Autodesk Fusion 360 part; units mm, degrees
(part 4 of 10)
sketch "草图11 (10)" plane through (0, 0, 36) normal (0, 0, 1) x (1, 0, 0) in component "LS_RemovableGrate"
  line L0 (60.3, 210) -> (159.7, 210)
  line L1 (159.7, 210) -> (159.7, 214)
  line L2 (159.7, 214) -> (60.3, 214)
  line L3 (60.3, 214) -> (60.3, 210)
  dimension "d1492" = 210
  dimension "d1493" = 99.4
  dimension "d1494" = 4
  constraint horizontal L0
  constraint vertical L1
  constraint horizontal L2
  constraint vertical L3
  measures "d1492" vertical distance of origin L0.start
  measures "d1493" horizontal distance of L0.start L0.end
  measures "d1494" vertical distance of L0.end L1.end
extrude "Drain slot 10''''" cut sketch "草图11 (10)" along normal blind 4 bodies 26 in component "LS_RemovableGrate"
ref_plane "工作平面12" through (0, 0, 36) normal (0, 0, 1) x (1, 0, 0) in component "LS_RemovableGrate"
sketch "草图12 (10)" plane through (0, 0, 36) normal (0, 0, 1) x (1, 0, 0) in component "LS_RemovableGrate"
  line L0 (60.3, 200) -> (159.7, 200)
  line L1 (159.7, 200) -> (159.7, 204)
  line L2 (159.7, 204) -> (60.3, 204)
  line L3 (60.3, 204) -> (60.3, 200)
  dimension "d1500" = 200
  dimension "d1501" = 99.4
  dimension "d1502" = 4
  constraint horizontal L0
  constraint vertical L1
  constraint horizontal L2
  constraint vertical L3
  measures "d1500" vertical distance of origin L0.start
  measures "d1501" horizontal distance of L0.start L0.end
  measures "d1502" vertical distance of L0.end L1.end
extrude "Drain slot 11''''" cut sketch "草图12 (10)" along normal blind 4 bodies 26 in component "LS_RemovableGrate"
ref_plane "工作平面13" through (0, 0, 36) normal (0, 0, 1) x (1, 0, 0) in component "LS_RemovableGrate"
sketch "草图13 (10)" plane through (0, 0, 36) normal (0, 0, 1) x (1, 0, 0) in component "LS_RemovableGrate"
  line L0 (60.3, 190) -> (159.7, 190)
  line L1 (159.7, 190) -> (159.7, 194)
  line L2 (159.7, 194) -> (60.3, 194)
  line L3 (60.3, 194) -> (60.3, 190)
  dimension "d1508" = 190
  dimension "d1509" = 99.4
  dimension "d1510" = 4
  constraint horizontal L0
  constraint vertical L1
  constraint horizontal L2
  constraint vertical L3
  measures "d1508" vertical distance of origin L0.start
  measures "d1509" horizontal distance of L0.start L0.end
  measures "d1510" vertical distance of L0.end L1.end
extrude "Drain slot 12''" cut sketch "草图13 (10)" along normal blind 4 bodies 26 in component "LS_RemovableGrate"
ref_plane "工作平面14" through (0, 0, 36) normal (0, 0, 1) x (1, 0, 0) in component "LS_RemovableGrate"
sketch "草图14 (8)" plane through (0, 0, 36) normal (0, 0, 1) x (1, 0, 0) in component "LS_RemovableGrate"
  line L0 (60.3, 180) -> (159.7, 180)
  line L1 (159.7, 180) -> (159.7, 184)
  line L2 (159.7, 184) -> (60.3, 184)
  line L3 (60.3, 184) -> (60.3, 180)
  dimension "d1516" = 180
  dimension "d1517" = 99.4
  dimension "d1518" = 4
  constraint horizontal L0
  constraint vertical L1
  constraint horizontal L2
  constraint vertical L3
  measures "d1516" vertical distance of origin L0.start
  measures "d1517" horizontal distance of L0.start L0.end
  measures "d1518" vertical distance of L0.end L1.end
extrude "Drain slot 13''" cut sketch "草图14 (8)" along normal blind 4 bodies 26 in component "LS_RemovableGrate"
ref_plane "工作平面15" through (0, 0, 36) normal (0, 0, 1) x (1, 0, 0) in component "LS_RemovableGrate"
sketch "草图15 (8)" plane through (0, 0, 36) normal (0, 0, 1) x (1, 0, 0) in component "LS_RemovableGrate"
  line L0 (60.3, 170) -> (159.7, 170)
  line L1 (159.7, 170) -> (159.7, 174)
  line L2 (159.7, 174) -> (60.3, 174)
  line L3 (60.3, 174) -> (60.3, 170)
  dimension "d1524" = 170
  dimension "d1525" = 99.4
  dimension "d1526" = 4
  constraint horizontal L0
  constraint vertical L1
  constraint horizontal L2
  constraint vertical L3
  measures "d1524" vertical distance of origin L0.start
  measures "d1525" horizontal distance of L0.start L0.end
  measures "d1526" vertical distance of L0.end L1.end
extrude "Drain slot 14'" cut sketch "草图15 (8)" along normal blind 4 bodies 26 in component "LS_RemovableGrate"
ref_plane "工作平面16" through (0, 0, 36) normal (0, 0, 1) x (1, 0, 0) in component "LS_RemovableGrate"
sketch "草图16 (2)" plane through (0, 0, 36) normal (0, 0, 1) x (1, 0, 0) in component "LS_RemovableGrate"
  line L0 (60.3, 160) -> (159.7, 160)
  line L1 (159.7, 160) -> (159.7, 164)
  line L2 (159.7, 164) -> (60.3, 164)
  line L3 (60.3, 164) -> (60.3, 160)
  dimension "d1532" = 160
  dimension "d1533" = 99.4
  dimension "d1534" = 4
  constraint horizontal L0
  constraint vertical L1
  constraint horizontal L2
  constraint vertical L3
  measures "d1532" vertical distance of origin L0.start
  measures "d1533" horizontal distance of L0.start L0.end
  measures "d1534" vertical distance of L0.end L1.end
extrude "Drain slot 15'" cut sketch "草图16 (2)" along normal blind 4 bodies 26 in component "LS_RemovableGrate"
ref_plane "工作平面17" through (0, 0, 36) normal (0, 0, 1) x (1, 0, 0) in component "LS_RemovableGrate"
sketch "草图17 (2)" plane through (0, 0, 36) normal (0, 0, 1) x (1, 0, 0) in component "LS_RemovableGrate"
  line L0 (162.7, 224) -> (167.7, 224)
  line L1 (167.7, 224) -> (167.7, 240)
  line L2 (167.7, 240) -> (162.7, 240)
  line L3 (162.7, 240) -> (162.7, 224)
  dimension "d1539" = 162.7
  dimension "d1540" = 224
  dimension "d1541" = 5
  dimension "d1542" = 16
  constraint horizontal L0
  constraint vertical L1
  constraint horizontal L2
  constraint vertical L3
  measures "d1539" horizontal distance of origin L0.start
  measures "d1540" vertical distance of origin L0.start
  measures "d1541" horizontal distance of L0.start L0.end
  measures "d1542" vertical distance of L0.end L1.end
extrude "Finger lift notch''''" cut sketch "草图17 (2)" along normal blind 4 bodies 26 in component "LS_RemovableGrate"
ref_plane "工作平面1" through (0, 0, 0) normal (0, 0, 1) x (1, 0, 0) in component "LS_Foot_00"
sketch "草图1 (27)" plane through (0, 0, 0) normal (0, 0, 1) x (1, 0, 0) in component "LS_Foot_00"
  line L0 (53, 303) -> (69, 303)
  line L1 (69, 303) -> (69, 319)
  line L2 (69, 319) -> (53, 319)
  line L3 (53, 319) -> (53, 303)
  dimension "d1547" = 53
  dimension "d1548" = 303
  dimension "d1549" = 16
  dimension "d1550" = 16
  constraint horizontal L0
  constraint vertical L1
  constraint horizontal L2
  constraint vertical L3
  measures "d1547" horizontal distance of origin L0.start
  measures "d1548" vertical distance of origin L0.start
  measures "d1549" horizontal distance of L0.start L0.end
  measures "d1550" vertical distance of L0.end L1.end
extrude "Foot base''''''''''''''''" add sketch "草图1 (27)" along normal blind 20 separate body makes body 27 in component "LS_Foot_00"
ref_plane "工作平面2" through (0, 0, 20) normal (0, 0, 1) x (1, 0, 0) in component "LS_Foot_00"
sketch "草图2 (27)" plane through (0, 0, 20) normal (0, 0, 1) x (1, 0, 0) in component "LS_Foot_00"
  line L0 (57, 307) -> (65, 307)
  line L1 (65, 307) -> (65, 315)
  line L2 (65, 315) -> (57, 315)
  line L3 (57, 315) -> (57, 307)
  dimension "d1555" = 57
  dimension "d1556" = 307
  dimension "d1557" = 8
  dimension "d1558" = 8
  constraint horizontal L0
  constraint vertical L1
  constraint horizontal L2
  constraint vertical L3
  measures "d1555" horizontal distance of origin L0.start
  measures "d1556" vertical distance of origin L0.start
  measures "d1557" horizontal distance of L0.start L0.end
  measures "d1558" vertical distance of L0.end L1.end
extrude "Locating peg''''''''''''''''" add sketch "草图2 (27)" along normal blind 1.5 bodies 27 in component "LS_Foot_00"
ref_plane "工作平面1" through (0, 0, 0) normal (0, 0, 1) x (1, 0, 0) in component "LS_Foot_01"
sketch "草图1 (28)" plane through (0, 0, 0) normal (0, 0, 1) x (1, 0, 0) in component "LS_Foot_01"
  line L0 (145, 303) -> (161, 303)
  line L1 (161, 303) -> (161, 319)
  line L2 (161, 319) -> (145, 319)
  line L3 (145, 319) -> (145, 303)
  dimension "d1563" = 145
  dimension "d1564" = 303
  dimension "d1565" = 16
  dimension "d1566" = 16
  constraint horizontal L0
  constraint vertical L1
  constraint horizontal L2
  constraint vertical L3
  measures "d1563" horizontal distance of origin L0.start
  measures "d1564" vertical distance of origin L0.start
  measures "d1565" horizontal distance of L0.start L0.end
  measures "d1566" vertical distance of L0.end L1.end
extrude "Foot base'''''''''''''''''" add sketch "草图1 (28)" along normal blind 20 separate body makes body 28 in component "LS_Foot_01"
ref_plane "工作平面2" through (0, 0, 20) normal (0, 0, 1) x (1, 0, 0) in component "LS_Foot_01"
sketch "草图2 (28)" plane through (0, 0, 20) normal (0, 0, 1) x (1, 0, 0) in component "LS_Foot_01"
  line L0 (149, 307) -> (157, 307)
  line L1 (157, 307) -> (157, 315)
  line L2 (157, 315) -> (149, 315)
  line L3 (149, 315) -> (149, 307)
  dimension "d1571" = 149
  dimension "d1572" = 307
  dimension "d1573" = 8
  dimension "d1574" = 8
  constraint horizontal L0
  constraint vertical L1
  constraint horizontal L2
  constraint vertical L3
  measures "d1571" horizontal distance of origin L0.start
  measures "d1572" vertical distance of origin L0.start
  measures "d1573" horizontal distance of L0.start L0.end
  measures "d1574" vertical distance of L0.end L1.end
extrude "Locating peg'''''''''''''''''" add sketch "草图2 (28)" along normal blind 1.5 bodies 28 in component "LS_Foot_01"
ref_plane "工作平面1" through (0, 0, 0) normal (0, 0, 1) x (1, 0, 0) in component "LS_Foot_10"
sketch "草图1 (29)" plane through (0, 0, 0) normal (0, 0, 1) x (1, 0, 0) in component "LS_Foot_10"
  line L0 (53, 145) -> (69, 145)
  line L1 (69, 145) -> (69, 161)
  line L2 (69, 161) -> (53, 161)
  line L3 (53, 161) -> (53, 145)
  dimension "d1579" = 53
  dimension "d1580" = 145
  dimension "d1581" = 16
  dimension "d1582" = 16
  constraint horizontal L0
  constraint vertical L1
  constraint horizontal L2
  constraint vertical L3
  measures "d1579" horizontal distance of origin L0.start
  measures "d1580" vertical distance of origin L0.start
  measures "d1581" horizontal distance of L0.start L0.end
  measures "d1582" vertical distance of L0.end L1.end
extrude "Foot base''''''''''''''''''" add sketch "草图1 (29)" along normal blind 20 separate body makes body 29 in component "LS_Foot_10"
ref_plane "工作平面2" through (0, 0, 20) normal (0, 0, 1) x (1, 0, 0) in component "LS_Foot_10"
sketch "草图2 (29)" plane through (0, 0, 20) normal (0, 0, 1) x (1, 0, 0) in component "LS_Foot_10"
  line L0 (57, 149) -> (65, 149)
  line L1 (65, 149) -> (65, 157)
  line L2 (65, 157) -> (57, 157)
  line L3 (57, 157) -> (57, 149)
  dimension "d1587" = 57
  dimension "d1588" = 149
  dimension "d1589" = 8
  dimension "d1590" = 8
  constraint horizontal L0
  constraint vertical L1
  constraint horizontal L2
  constraint vertical L3
  measures "d1587" horizontal distance of origin L0.start
  measures "d1588" vertical distance of origin L0.start
  measures "d1589" horizontal distance of L0.start L0.end
  measures "d1590" vertical distance of L0.end L1.end
extrude "Locating peg''''''''''''''''''" add sketch "草图2 (29)" along normal blind 1.5 bodies 29 in component "LS_Foot_10"
ref_plane "工作平面1" through (0, 0, 0) normal (0, 0, 1) x (1, 0, 0) in component "LS_Foot_11"
sketch "草图1 (30)" plane through (0, 0, 0) normal (0, 0, 1) x (1, 0, 0) in component "LS_Foot_11"
  line L0 (145, 145) -> (161, 145)
  line L1 (161, 145) -> (161, 161)
  line L2 (161, 161) -> (145, 161)
  line L3 (145, 161) -> (145, 145)
  dimension "d1595" = 145
  dimension "d1596" = 145
  dimension "d1597" = 16
  dimension "d1598" = 16
  constraint horizontal L0
  constraint vertical L1
  constraint horizontal L2
  constraint vertical L3
  measures "d1595" horizontal distance of origin L0.start
  measures "d1596" vertical distance of origin L0.start
  measures "d1597" horizontal distance of L0.start L0.end
  measures "d1598" vertical distance of L0.end L1.end
extrude "Foot base'''''''''''''''''''" add sketch "草图1 (30)" along normal blind 20 separate body makes body 30 in component "LS_Foot_11"
ref_plane "工作平面2" through (0, 0, 20) normal (0, 0, 1) x (1, 0, 0) in component "LS_Foot_11"
sketch "草图2 (30)" plane through (0, 0, 20) normal (0, 0, 1) x (1, 0, 0) in component "LS_Foot_11"
  line L0 (149, 149) -> (157, 149)
  line L1 (157, 149) -> (157, 157)
  line L2 (157, 157) -> (149, 157)
  line L3 (149, 157) -> (149, 149)
  dimension "d1603" = 149
  dimension "d1604" = 149
  dimension "d1605" = 8
  dimension "d1606" = 8
  constraint horizontal L0
  constraint vertical L1
  constraint horizontal L2
  constraint vertical L3
  measures "d1603" horizontal distance of origin L0.start
  measures "d1604" vertical distance of origin L0.start
  measures "d1605" horizontal distance of L0.start L0.end
  measures "d1606" vertical distance of L0.end L1.end
extrude "Locating peg'''''''''''''''''''" add sketch "草图2 (30)" along normal blind 1.5 bodies 30 in component "LS_Foot_11"
ref_plane "工作平面1" through (0, 0, 20) normal (0, 0, 1) x (1, 0, 0) in component "RS_Integrated"
sketch "草图1 (31)" plane through (0, 0, 20) normal (0, 0, 1) x (1, 0, 0) in component "RS_Integrated"
  line L0 (770, 142) -> (860, 142)
  line L1 (860, 142) -> (860, 322)
  line L2 (860, 322) -> (770, 322)
  line L3 (770, 322) -> (770, 142)
  dimension "d1611" = 770
  dimension "d1612" = 142
  dimension "d1613" = 90
  dimension "d1614" = 180
  constraint horizontal L0
  constraint vertical L1
  constraint horizontal L2
  constraint vertical L3
  measures "d1611" horizontal distance of origin L0.start
  measures "d1612" vertical distance of origin L0.start
  measures "d1613" horizontal distance of L0.start L0.end
  measures "d1614" vertical distance of L0.end L1.end
extrude "Pan blank'''''" add sketch "草图1 (31)" along normal blind 20 separate body makes body 31 in component "RS_Integrated"
fillet "Outside corner rounds'''''" radius 3 4 edges at (770, 322, 30) (860, 322, 30) (860, 142, 30) (770, 142, 30) on bodies 31 in component "RS_Integrated"
ref_plane "工作平面2" through (0, 145, 0) normal (0, 1, 0) x (0, 0, 1) in component "RS_Integrated"
sketch "草图2 (31)" plane through (0, 145, 0) normal (0, 1, 0) x (1, 0, 0) in component "RS_Integrated"
  line L0 (857, -30.8318) -> (773, -24.958)
  line L1 (773, -24.958) -> (773, -41)
  line L2 (773, -41) -> (857, -41)
  line L3 (857, -41) -> (857, -30.8318)
  dimension "d1621" = 857
  dimension "d1622" = 30.8318
  dimension "d1623" = 773
  dimension "d1624" = 24.958
  dimension "d1625" = 41
  constraint vertical L1
  constraint horizontal L2
  constraint vertical L3
  measures "d1621" horizontal distance of origin L0.start
  measures "d1622" vertical distance of origin L0.start
  measures "d1623" horizontal distance of origin L0.end
  measures "d1624" vertical distance of origin L0.end
  measures "d1625" vertical distance of origin L1.end
extrude "Sloped catch cavity'''''" cut sketch "草图2 (31)" along normal blind 174 bodies 31 in component "RS_Integrated"
ref_plane "工作平面3" through (0, 215, 0) normal (0, 1, 0) x (0, 0, 1) in component "RS_Integrated"
sketch "草图3 (11)" plane through (0, 215, 0) normal (0, 1, 0) x (1, 0, 0) in component "RS_Integrated"
  line L0 (773, -20) -> (745, -20)
  line L1 (745, -20) -> (745, -23)
  line L2 (745, -23) -> (773, -24.958)
  line L3 (773, -24.958) -> (773, -20)
  dimension "d1630" = 773
  dimension "d1632" = 745
  dimension "d1633" = 23
  dimension "d1634" = 24.958
  constraint horizontal L0
  constraint vertical L1
  constraint vertical L3
  measures "d1630" horizontal distance of origin L0.start
  measures "d1632" horizontal distance of origin L0.end
  measures "d1633" vertical distance of origin L1.end
  measures "d1634" vertical distance of origin L2.end
extrude "Drain tongue floor'''''" add sketch "草图3 (11)" along normal blind 34 bodies 31 in component "RS_Integrated"
ref_plane "工作平面4" through (0, 215, 0) normal (0, 1, 0) x (0, 0, 1) in component "RS_Integrated"
sketch "草图4 (11)" plane through (0, 215, 0) normal (0, 1, 0) x (1, 0, 0) in component "RS_Integrated"
  line L0 (773, -20) -> (745, -20)
  line L1 (745, -20) -> (745, -29)
  line L2 (745, -29) -> (773, -30.958)
  line L3 (773, -30.958) -> (773, -20)
  dimension "d1639" = 773
  dimension "d1641" = 745
  dimension "d1642" = 29
  dimension "d1643" = 30.958
  constraint horizontal L0
  constraint vertical L1
  constraint vertical L3
  measures "d1639" horizontal distance of origin L0.start
  measures "d1641" horizontal distance of origin L0.end
  measures "d1642" vertical distance of origin L1.end
  measures "d1643" vertical distance of origin L2.end
extrude "Tongue side rail'''''" add sketch "草图4 (11)" along normal blind 3 bodies 31 in component "RS_Integrated"
ref_plane "工作平面5" through (0, 246, 0) normal (0, 1, 0) x (0, 0, 1) in component "RS_Integrated"
sketch "草图5 (11)" plane through (0, 246, 0) normal (0, 1, 0) x (1, 0, 0) in component "RS_Integrated"
  line L0 (773, -20) -> (745, -20)
  line L1 (745, -20) -> (745, -29)
  line L2 (745, -29) -> (773, -30.958)
  line L3 (773, -30.958) -> (773, -20)
  dimension "d1648" = 773
  dimension "d1650" = 745
  dimension "d1651" = 29
  dimension "d1652" = 30.958
  constraint horizontal L0
  constraint vertical L1
  constraint vertical L3
  measures "d1648" horizontal distance of origin L0.start
  measures "d1650" horizontal distance of origin L0.end
  measures "d1651" vertical distance of origin L1.end
  measures "d1652" vertical distance of origin L2.end
extrude "Tongue side rail (1)'''''" add sketch "草图5 (11)" along normal blind 3 bodies 31 in component "RS_Integrated"
ref_plane "工作平面6" through (0, 218, 0) normal (0, 1, 0) x (0, 0, 1) in component "RS_Integrated"
sketch "草图6 (11)" plane through (0, 218, 0) normal (0, 1, 0) x (1, 0, 0) in component "RS_Integrated"
  line L0 (773, -24.958) -> (745, -23)
  line L1 (745, -23) -> (745, -41)
  line L2 (745, -41) -> (773, -41)
  line L3 (773, -41) -> (773, -24.958)
  dimension "d1657" = 773
  dimension "d1658" = 24.958
  dimension "d1659" = 745
  dimension "d1660" = 23
  dimension "d1661" = 41
  constraint vertical L1
  constraint horizontal L2
  constraint vertical L3
  measures "d1657" horizontal distance of origin L0.start
  measures "d1658" vertical distance of origin L0.start
  measures "d1659" horizontal distance of origin L0.end
  measures "d1660" vertical distance of origin L0.end
  measures "d1661" vertical distance of origin L1.end
extrude "Open drain mouth'''''" cut sketch "草图6 (11)" along normal blind 28 bodies 31 in component "RS_Integrated"
ref_plane "工作平面7" through (0, 0, 20) normal (0, 0, 1) x (1, 0, 0) in component "RS_Integrated"
sketch "草图7 (11)" plane through (0, 0, 20) normal (0, 0, 1) x (1, 0, 0) in component "RS_Integrated"
  line L0 (845, 145) -> (857, 145)
  line L1 (857, 145) -> (857, 157)
  line L2 (857, 157) -> (845, 157)
  line L3 (845, 157) -> (845, 145)
  dimension "d1666" = 845
  dimension "d1668" = 12
  dimension "d1669" = 12
  constraint horizontal L0
  constraint vertical L1
  constraint horizontal L2
  constraint vertical L3
  measures "d1666" horizontal distance of origin L0.start
  measures "d1668" horizontal distance of L0.start L0.end
  measures "d1669" vertical distance of L0.end L1.end
extrude "Grate seat 00'''''" add sketch "草图7 (11)" along normal blind 16 bodies 31 in component "RS_Integrated"
ref_plane "工作平面8" through (0, 0, 20) normal (0, 0, 1) x (1, 0, 0) in component "RS_Integrated"
sketch "草图8 (11)" plane through (0, 0, 20) normal (0, 0, 1) x (1, 0, 0) in component "RS_Integrated"
  line L0 (773, 145) -> (785, 145)
  line L1 (785, 145) -> (785, 157)
  line L2 (785, 157) -> (773, 157)
  line L3 (773, 157) -> (773, 145)
  dimension "d1674" = 773
  dimension "d1676" = 12
  dimension "d1677" = 12
  constraint horizontal L0
  constraint vertical L1
  constraint horizontal L2
  constraint vertical L3
  measures "d1674" horizontal distance of origin L0.start
  measures "d1676" horizontal distance of L0.start L0.end
  measures "d1677" vertical distance of L0.end L1.end
extrude "Grate seat 01'''''" add sketch "草图8 (11)" along normal blind 16 bodies 31 in component "RS_Integrated"
ref_plane "工作平面9" through (0, 0, 20) normal (0, 0, 1) x (1, 0, 0) in component "RS_Integrated"
sketch "草图9 (11)" plane through (0, 0, 20) normal (0, 0, 1) x (1, 0, 0) in component "RS_Integrated"
  line L0 (845, 307) -> (857, 307)
  line L1 (857, 307) -> (857, 319)
  line L2 (857, 319) -> (845, 319)
  line L3 (845, 319) -> (845, 307)
  dimension "d1682" = 845
  dimension "d1683" = 307
  dimension "d1684" = 12
  dimension "d1685" = 12
  constraint horizontal L0
  constraint vertical L1
  constraint horizontal L2
  constraint vertical L3
  measures "d1682" horizontal distance of origin L0.start
  measures "d1683" vertical distance of origin L0.start
  measures "d1684" horizontal distance of L0.start L0.end
  measures "d1685" vertical distance of L0.end L1.end
extrude "Grate seat 10'''''" add sketch "草图9 (11)" along normal blind 16 bodies 31 in component "RS_Integrated"
ref_plane "工作平面10" through (0, 0, 20) normal (0, 0, 1) x (1, 0, 0) in component "RS_Integrated"
sketch "草图10 (11)" plane through (0, 0, 20) normal (0, 0, 1) x (1, 0, 0) in component "RS_Integrated"
  line L0 (773, 307) -> (785, 307)
  line L1 (785, 307) -> (785, 319)
  line L2 (785, 319) -> (773, 319)
  line L3 (773, 319) -> (773, 307)
  dimension "d1690" = 773
  dimension "d1691" = 307
  dimension "d1692" = 12
  dimension "d1693" = 12
  constraint horizontal L0
  constraint vertical L1
  constraint horizontal L2
  constraint vertical L3
  measures "d1690" horizontal distance of origin L0.start
  measures "d1691" vertical distance of origin L0.start
  measures "d1692" horizontal distance of L0.start L0.end
  measures "d1693" vertical distance of L0.end L1.end
extrude "Grate seat 11'''''" add sketch "草图10 (11)" along normal blind 16 bodies 31 in component "RS_Integrated"
ref_plane "工作平面11" through (0, 215, 0) normal (0, 1, 0) x (0, 0, 1) in component "RS_Integrated"
sketch "草图11 (11)" plane through (0, 215, 0) normal (0, 1, 0) x (1, 0, 0) in component "RS_Integrated"
  line L0 (747, -19.8) -> (746, -19.8)
  line L1 (746, -19.8) -> (746, -20.6)
  line L2 (746, -20.6) -> (747, -20.6)
  line L3 (747, -20.6) -> (747, -19.8)
  dimension "d1698" = 747
  dimension "d1699" = 19.8
  dimension "d1700" = 746
  dimension "d1701" = 20.6
  constraint horizontal L0
  constraint vertical L1
  constraint horizontal L2
  constraint vertical L3
  measures "d1698" horizontal distance of origin L0.start
  measures "d1699" vertical distance of origin L0.start
  measures "d1700" horizontal distance of origin L0.end
  measures "d1701" vertical distance of origin L1.end
extrude "Drip break underside groove'''''" cut sketch "草图11 (11)" along normal blind 34 bodies 31 in component "RS_Integrated"
ref_plane "工作平面12" through (0, 0, 20) normal (0, 0, 1) x (1, 0, 0) in component "RS_Integrated"
sketch "草图12 (11)" plane through (0, 0, 20) normal (0, 0, 1) x (1, 0, 0) in component "RS_Integrated"
  line L0 (844.75, 148.75) -> (853.25, 148.75)
  line L1 (853.25, 148.75) -> (853.25, 157.25)
  line L2 (853.25, 157.25) -> (844.75, 157.25)
  line L3 (844.75, 157.25) -> (844.75, 148.75)
  dimension "d1706" = 844.75
  dimension "d1707" = 148.75
  dimension "d1708" = 8.5
  dimension "d1709" = 8.5
  constraint horizontal L0
  constraint vertical L1
  constraint horizontal L2
  constraint vertical L3
  measures "d1706" horizontal distance of origin L0.start
  measures "d1707" vertical distance of origin L0.start
  measures "d1708" horizontal distance of L0.start L0.end
  measures "d1709" vertical distance of L0.end L1.end
extrude "Foot socket 00'''''" cut sketch "草图12 (11)" along normal blind 1.8 bodies 31 in component "RS_Integrated"
ref_plane "工作平面13" through (0, 0, 20) normal (0, 0, 1) x (1, 0, 0) in component "RS_Integrated"
sketch "草图13 (11)" plane through (0, 0, 20) normal (0, 0, 1) x (1, 0, 0) in component "RS_Integrated"
  line L0 (782.75, 148.75) -> (791.25, 148.75)
  line L1 (791.25, 148.75) -> (791.25, 157.25)
  line L2 (791.25, 157.25) -> (782.75, 157.25)
  line L3 (782.75, 157.25) -> (782.75, 148.75)
  dimension "d1714" = 782.75
  dimension "d1715" = 148.75
  dimension "d1716" = 8.5
  dimension "d1717" = 8.5
  constraint horizontal L0
  constraint vertical L1
  constraint horizontal L2
  constraint vertical L3
  measures "d1714" horizontal distance of origin L0.start
  measures "d1715" vertical distance of origin L0.start
  measures "d1716" horizontal distance of L0.start L0.end
  measures "d1717" vertical distance of L0.end L1.end
extrude "Foot socket 01'''''" cut sketch "草图13 (11)" along normal blind 1.8 bodies 31 in component "RS_Integrated"
ref_plane "工作平面14" through (0, 0, 20) normal (0, 0, 1) x (1, 0, 0) in component "RS_Integrated"
sketch "草图14 (9)" plane through (0, 0, 20) normal (0, 0, 1) x (1, 0, 0) in component "RS_Integrated"
  line L0 (844.75, 306.75) -> (853.25, 306.75)
  line L1 (853.25, 306.75) -> (853.25, 315.25)
  line L2 (853.25, 315.25) -> (844.75, 315.25)
  line L3 (844.75, 315.25) -> (844.75, 306.75)
  dimension "d1722" = 844.75
  dimension "d1723" = 306.75
  dimension "d1724" = 8.5
  dimension "d1725" = 8.5
  constraint horizontal L0
  constraint vertical L1
  constraint horizontal L2
  constraint vertical L3
  measures "d1722" horizontal distance of origin L0.start
  measures "d1723" vertical distance of origin L0.start
  measures "d1724" horizontal distance of L0.start L0.end
  measures "d1725" vertical distance of L0.end L1.end
extrude "Foot socket 10'''''" cut sketch "草图14 (9)" along normal blind 1.8 bodies 31 in component "RS_Integrated"
ref_plane "工作平面15" through (0, 0, 20) normal (0, 0, 1) x (1, 0, 0) in component "RS_Integrated"
sketch "草图15 (9)" plane through (0, 0, 20) normal (0, 0, 1) x (1, 0, 0) in component "RS_Integrated"
  line L0 (782.75, 306.75) -> (791.25, 306.75)
  line L1 (791.25, 306.75) -> (791.25, 315.25)
  line L2 (791.25, 315.25) -> (782.75, 315.25)
  line L3 (782.75, 315.25) -> (782.75, 306.75)
  dimension "d1730" = 782.75
  dimension "d1731" = 306.75
  dimension "d1732" = 8.5
  dimension "d1733" = 8.5
  constraint horizontal L0
  constraint vertical L1
  constraint horizontal L2
  constraint vertical L3
  measures "d1730" horizontal distance of origin L0.start
  measures "d1731" vertical distance of origin L0.start
  measures "d1732" horizontal distance of L0.start L0.end
  measures "d1733" vertical distance of L0.end L1.end
extrude "Foot socket 11'''''" cut sketch "草图15 (9)" along normal blind 1.8 bodies 31 in component "RS_Integrated"
ref_plane "工作平面1" through (0, 0, 36) normal (0, 0, 1) x (1, 0, 0) in component "RS_RemovableGrate"
sketch "草图1 (32)" plane through (0, 0, 36) normal (0, 0, 1) x (1, 0, 0) in component "RS_RemovableGrate"
  line L0 (773.3, 145.3) -> (856.7, 145.3)
  line L1 (856.7, 145.3) -> (856.7, 318.7)
  line L2 (856.7, 318.7) -> (773.3, 318.7)
  line L3 (773.3, 318.7) -> (773.3, 145.3)
  dimension "d1738" = 773.3
  dimension "d1740" = 83.4
  dimension "d1741" = 173.4
  constraint horizontal L0
  constraint vertical L1
  constraint horizontal L2
  constraint vertical L3
  measures "d1738" horizontal distance of origin L0.start
  measures "d1740" horizontal distance of L0.start L0.end
  measures "d1741" vertical distance of L0.end L1.end
extrude "Horizontal removable deck'''''" add sketch "草图1 (32)" along normal blind 4 separate body makes body 32 in component "RS_RemovableGrate"
ref_plane "工作平面2" through (0, 0, 36) normal (0, 0, 1) x (1, 0, 0) in component "RS_RemovableGrate"
sketch "草图2 (32)" plane through (0, 0, 36) normal (0, 0, 1) x (1, 0, 0) in component "RS_RemovableGrate"
  line L0 (780.3, 160) -> (849.7, 160)
  line L1 (849.7, 160) -> (849.7, 164)
  line L2 (849.7, 164) -> (780.3, 164)
  line L3 (780.3, 164) -> (780.3, 160)
  dimension "d1746" = 780.3
  dimension "d1747" = 160
  dimension "d1748" = 69.4
  dimension "d1749" = 4
  constraint horizontal L0
  constraint vertical L1
  constraint horizontal L2
  constraint vertical L3
  measures "d1746" horizontal distance of origin L0.start
  measures "d1747" vertical distance of origin L0.start
  measures "d1748" horizontal distance of L0.start L0.end
  measures "d1749" vertical distance of L0.end L1.end
extrude "Drain slot 1'''''" cut sketch "草图2 (32)" along normal blind 4 bodies 32 in component "RS_RemovableGrate"
ref_plane "工作平面3" through (0, 0, 36) normal (0, 0, 1) x (1, 0, 0) in component "RS_RemovableGrate"
sketch "草图3 (12)" plane through (0, 0, 36) normal (0, 0, 1) x (1, 0, 0) in component "RS_RemovableGrate"
  line L0 (780.3, 170) -> (849.7, 170)
  line L1 (849.7, 170) -> (849.7, 174)
  line L2 (849.7, 174) -> (780.3, 174)
  line L3 (780.3, 174) -> (780.3, 170)
  dimension "d1754" = 780.3
  dimension "d1755" = 170
  dimension "d1756" = 69.4
  dimension "d1757" = 4
  constraint horizontal L0
  constraint vertical L1
  constraint horizontal L2
  constraint vertical L3
  measures "d1754" horizontal distance of origin L0.start
  measures "d1755" vertical distance of origin L0.start
  measures "d1756" horizontal distance of L0.start L0.end
  measures "d1757" vertical distance of L0.end L1.end
extrude "Drain slot 2'''''" cut sketch "草图3 (12)" along normal blind 4 bodies 32 in component "RS_RemovableGrate"
ref_plane "工作平面4" through (0, 0, 36) normal (0, 0, 1) x (1, 0, 0) in component "RS_RemovableGrate"
sketch "草图4 (12)" plane through (0, 0, 36) normal (0, 0, 1) x (1, 0, 0) in component "RS_RemovableGrate"
  line L0 (780.3, 180) -> (849.7, 180)
  line L1 (849.7, 180) -> (849.7, 184)
  line L2 (849.7, 184) -> (780.3, 184)
  line L3 (780.3, 184) -> (780.3, 180)
  dimension "d1762" = 780.3
  dimension "d1763" = 180
  dimension "d1764" = 69.4
  dimension "d1765" = 4
  constraint horizontal L0
  constraint vertical L1
  constraint horizontal L2
  constraint vertical L3
  measures "d1762" horizontal distance of origin L0.start
  measures "d1763" vertical distance of origin L0.start
  measures "d1764" horizontal distance of L0.start L0.end
  measures "d1765" vertical distance of L0.end L1.end
extrude "Drain slot 3'''''" cut sketch "草图4 (12)" along normal blind 4 bodies 32 in component "RS_RemovableGrate"
ref_plane "工作平面5" through (0, 0, 36) normal (0, 0, 1) x (1, 0, 0) in component "RS_RemovableGrate"
sketch "草图5 (12)" plane through (0, 0, 36) normal (0, 0, 1) x (1, 0, 0) in component "RS_RemovableGrate"
  line L0 (780.3, 190) -> (849.7, 190)
  line L1 (849.7, 190) -> (849.7, 194)
  line L2 (849.7, 194) -> (780.3, 194)
  line L3 (780.3, 194) -> (780.3, 190)
  dimension "d1770" = 780.3
  dimension "d1771" = 190
  dimension "d1772" = 69.4
  dimension "d1773" = 4
  constraint horizontal L0
  constraint vertical L1
  constraint horizontal L2
  constraint vertical L3
  measures "d1770" horizontal distance of origin L0.start
  measures "d1771" vertical distance of origin L0.start
  measures "d1772" horizontal distance of L0.start L0.end
  measures "d1773" vertical distance of L0.end L1.end
extrude "Drain slot 4'''''" cut sketch "草图5 (12)" along normal blind 4 bodies 32 in component "RS_RemovableGrate"
ref_plane "工作平面6" through (0, 0, 36) normal (0, 0, 1) x (1, 0, 0) in component "RS_RemovableGrate"
sketch "草图6 (12)" plane through (0, 0, 36) normal (0, 0, 1) x (1, 0, 0) in component "RS_RemovableGrate"
  line L0 (780.3, 200) -> (849.7, 200)
  line L1 (849.7, 200) -> (849.7, 204)
  line L2 (849.7, 204) -> (780.3, 204)
  line L3 (780.3, 204) -> (780.3, 200)
  dimension "d1778" = 780.3
  dimension "d1779" = 200
  dimension "d1780" = 69.4
  dimension "d1781" = 4
  constraint horizontal L0
  constraint vertical L1
  constraint horizontal L2
  constraint vertical L3
  measures "d1778" horizontal distance of origin L0.start
  measures "d1779" vertical distance of origin L0.start
  measures "d1780" horizontal distance of L0.start L0.end
  measures "d1781" vertical distance of L0.end L1.end
extrude "Drain slot 5'''''" cut sketch "草图6 (12)" along normal blind 4 bodies 32 in component "RS_RemovableGrate"
ref_plane "工作平面7" through (0, 0, 36) normal (0, 0, 1) x (1, 0, 0) in component "RS_RemovableGrate"
sketch "草图7 (12)" plane through (0, 0, 36) normal (0, 0, 1) x (1, 0, 0) in component "RS_RemovableGrate"
  line L0 (780.3, 210) -> (849.7, 210)
  line L1 (849.7, 210) -> (849.7, 214)
  line L2 (849.7, 214) -> (780.3, 214)
  line L3 (780.3, 214) -> (780.3, 210)
  dimension "d1786" = 780.3
  dimension "d1787" = 210
  dimension "d1788" = 69.4
  dimension "d1789" = 4
  constraint horizontal L0
  constraint vertical L1
  constraint horizontal L2
  constraint vertical L3
  measures "d1786" horizontal distance of origin L0.start
  measures "d1787" vertical distance of origin L0.start
  measures "d1788" horizontal distance of L0.start L0.end
  measures "d1789" vertical distance of L0.end L1.end
extrude "Drain slot 6'''''" cut sketch "草图7 (12)" along normal blind 4 bodies 32 in component "RS_RemovableGrate"
ref_plane "工作平面8" through (0, 0, 36) normal (0, 0, 1) x (1, 0, 0) in component "RS_RemovableGrate"
sketch "草图8 (12)" plane through (0, 0, 36) normal (0, 0, 1) x (1, 0, 0) in component "RS_RemovableGrate"
  line L0 (780.3, 220) -> (849.7, 220)
  line L1 (849.7, 220) -> (849.7, 224)
  line L2 (849.7, 224) -> (780.3, 224)
  line L3 (780.3, 224) -> (780.3, 220)
  dimension "d1794" = 780.3
  dimension "d1795" = 220
  dimension "d1796" = 69.4
  dimension "d1797" = 4
  constraint horizontal L0
  constraint vertical L1
  constraint horizontal L2
  constraint vertical L3
  measures "d1794" horizontal distance of origin L0.start
  measures "d1795" vertical distance of origin L0.start
  measures "d1796" horizontal distance of L0.start L0.end
  measures "d1797" vertical distance of L0.end L1.end
extrude "Drain slot 7'''''" cut sketch "草图8 (12)" along normal blind 4 bodies 32 in component "RS_RemovableGrate"
ref_plane "工作平面9" through (0, 0, 36) normal (0, 0, 1) x (1, 0, 0) in component "RS_RemovableGrate"
sketch "草图9 (12)" plane through (0, 0, 36) normal (0, 0, 1) x (1, 0, 0) in component "RS_RemovableGrate"
  line L0 (780.3, 230) -> (849.7, 230)
  line L1 (849.7, 230) -> (849.7, 234)
  line L2 (849.7, 234) -> (780.3, 234)
  line L3 (780.3, 234) -> (780.3, 230)
  dimension "d1802" = 780.3
  dimension "d1803" = 230
  dimension "d1804" = 69.4
  dimension "d1805" = 4
  constraint horizontal L0
  constraint vertical L1
  constraint horizontal L2
  constraint vertical L3
  measures "d1802" horizontal distance of origin L0.start
  measures "d1803" vertical distance of origin L0.start
  measures "d1804" horizontal distance of L0.start L0.end
  measures "d1805" vertical distance of L0.end L1.end
extrude "Drain slot 8'''''" cut sketch "草图9 (12)" along normal blind 4 bodies 32 in component "RS_RemovableGrate"
ref_plane "工作平面10" through (0, 0, 36) normal (0, 0, 1) x (1, 0, 0) in component "RS_RemovableGrate"
sketch "草图10 (12)" plane through (0, 0, 36) normal (0, 0, 1) x (1, 0, 0) in component "RS_RemovableGrate"
  line L0 (780.3, 240) -> (849.7, 240)
  line L1 (849.7, 240) -> (849.7, 244)
  line L2 (849.7, 244) -> (780.3, 244)
  line L3 (780.3, 244) -> (780.3, 240)
  dimension "d1810" = 780.3
  dimension "d1811" = 240
  dimension "d1812" = 69.4
  dimension "d1813" = 4
  constraint horizontal L0
  constraint vertical L1
  constraint horizontal L2
  constraint vertical L3
  measures "d1810" horizontal distance of origin L0.start
  measures "d1811" vertical distance of origin L0.start
  measures "d1812" horizontal distance of L0.start L0.end
  measures "d1813" vertical distance of L0.end L1.end
extrude "Drain slot 9'''''" cut sketch "草图10 (12)" along normal blind 4 bodies 32 in component "RS_RemovableGrate"
ref_plane "工作平面11" through (0, 0, 36) normal (0, 0, 1) x (1, 0, 0) in component "RS_RemovableGrate"
sketch "草图11 (12)" plane through (0, 0, 36) normal (0, 0, 1) x (1, 0, 0) in component "RS_RemovableGrate"
  line L0 (780.3, 250) -> (849.7, 250)
  line L1 (849.7, 250) -> (849.7, 254)
  line L2 (849.7, 254) -> (780.3, 254)
  line L3 (780.3, 254) -> (780.3, 250)
  dimension "d1818" = 780.3
  dimension "d1819" = 250
  dimension "d1820" = 69.4
  dimension "d1821" = 4
  constraint horizontal L0
  constraint vertical L1
  constraint horizontal L2
  constraint vertical L3
  measures "d1818" horizontal distance of origin L0.start
  measures "d1819" vertical distance of origin L0.start
  measures "d1820" horizontal distance of L0.start L0.end
  measures "d1821" vertical distance of L0.end L1.end
extrude "Drain slot 10'''''" cut sketch "草图11 (12)" along normal blind 4 bodies 32 in component "RS_RemovableGrate"
ref_plane "工作平面12" through (0, 0, 36) normal (0, 0, 1) x (1, 0, 0) in component "RS_RemovableGrate"
sketch "草图12 (12)" plane through (0, 0, 36) normal (0, 0, 1) x (1, 0, 0) in component "RS_RemovableGrate"
  line L0 (780.3, 260) -> (849.7, 260)
  line L1 (849.7, 260) -> (849.7, 264)
  line L2 (849.7, 264) -> (780.3, 264)
  line L3 (780.3, 264) -> (780.3, 260)
  dimension "d1826" = 780.3
  dimension "d1827" = 260
  dimension "d1828" = 69.4
  dimension "d1829" = 4
  constraint horizontal L0
  constraint vertical L1
  constraint horizontal L2
  constraint vertical L3
  measures "d1826" horizontal distance of origin L0.start
  measures "d1827" vertical distance of origin L0.start
  measures "d1828" horizontal distance of L0.start L0.end
  measures "d1829" vertical distance of L0.end L1.end
extrude "Drain slot 11'''''" cut sketch "草图12 (12)" along normal blind 4 bodies 32 in component "RS_RemovableGrate"
ref_plane "工作平面13" through (0, 0, 36) normal (0, 0, 1) x (1, 0, 0) in component "RS_RemovableGrate"
sketch "草图13 (12)" plane through (0, 0, 36) normal (0, 0, 1) x (1, 0, 0) in component "RS_RemovableGrate"
  line L0 (780.3, 270) -> (849.7, 270)
  line L1 (849.7, 270) -> (849.7, 274)
  line L2 (849.7, 274) -> (780.3, 274)
  line L3 (780.3, 274) -> (780.3, 270)
  dimension "d1834" = 780.3
  dimension "d1835" = 270
  dimension "d1836" = 69.4
  dimension "d1837" = 4
  constraint horizontal L0
  constraint vertical L1
  constraint horizontal L2
  constraint vertical L3
  measures "d1834" horizontal distance of origin L0.start
  measures "d1835" vertical distance of origin L0.start
  measures "d1836" horizontal distance of L0.start L0.end
  measures "d1837" vertical distance of L0.end L1.end
extrude "Drain slot 12'''" cut sketch "草图13 (12)" along normal blind 4 bodies 32 in component "RS_RemovableGrate"
ref_plane "工作平面14" through (0, 0, 36) normal (0, 0, 1) x (1, 0, 0) in component "RS_RemovableGrate"
sketch "草图14 (10)" plane through (0, 0, 36) normal (0, 0, 1) x (1, 0, 0) in component "RS_RemovableGrate"
  line L0 (780.3, 280) -> (849.7, 280)
  line L1 (849.7, 280) -> (849.7, 284)
  line L2 (849.7, 284) -> (780.3, 284)
  line L3 (780.3, 284) -> (780.3, 280)
  dimension "d1842" = 780.3
  dimension "d1843" = 280
  dimension "d1844" = 69.4
  dimension "d1845" = 4
  constraint horizontal L0
  constraint vertical L1
  constraint horizontal L2
  constraint vertical L3
  measures "d1842" horizontal distance of origin L0.start
  measures "d1843" vertical distance of origin L0.start
  measures "d1844" horizontal distance of L0.start L0.end
  measures "d1845" vertical distance of L0.end L1.end
extrude "Drain slot 13'''" cut sketch "草图14 (10)" along normal blind 4 bodies 32 in component "RS_RemovableGrate"
ref_plane "工作平面15" through (0, 0, 36) normal (0, 0, 1) x (1, 0, 0) in component "RS_RemovableGrate"
sketch "草图15 (10)" plane through (0, 0, 36) normal (0, 0, 1) x (1, 0, 0) in component "RS_RemovableGrate"
  line L0 (780.3, 290) -> (849.7, 290)
  line L1 (849.7, 290) -> (849.7, 294)
  line L2 (849.7, 294) -> (780.3, 294)
  line L3 (780.3, 294) -> (780.3, 290)
  dimension "d1850" = 780.3
  dimension "d1851" = 290
  dimension "d1852" = 69.4
  dimension "d1853" = 4
  constraint horizontal L0
  constraint vertical L1
  constraint horizontal L2
  constraint vertical L3
  measures "d1850" horizontal distance of origin L0.start
  measures "d1851" vertical distance of origin L0.start
  measures "d1852" horizontal distance of L0.start L0.end
  measures "d1853" vertical distance of L0.end L1.end
extrude "Drain slot 14''" cut sketch "草图15 (10)" along normal blind 4 bodies 32 in component "RS_RemovableGrate"
ref_plane "工作平面16" through (0, 0, 36) normal (0, 0, 1) x (1, 0, 0) in component "RS_RemovableGrate"
sketch "草图16 (3)" plane through (0, 0, 36) normal (0, 0, 1) x (1, 0, 0) in component "RS_RemovableGrate"
  line L0 (780.3, 300) -> (849.7, 300)
  line L1 (849.7, 300) -> (849.7, 304)
  line L2 (849.7, 304) -> (780.3, 304)
  line L3 (780.3, 304) -> (780.3, 300)
  dimension "d1858" = 780.3
  dimension "d1859" = 300
  dimension "d1860" = 69.4
  dimension "d1861" = 4
  constraint horizontal L0
  constraint vertical L1
  constraint horizontal L2
  constraint vertical L3
  measures "d1858" horizontal distance of origin L0.start
  measures "d1859" vertical distance of origin L0.start
  measures "d1860" horizontal distance of L0.start L0.end
  measures "d1861" vertical distance of L0.end L1.end
extrude "Drain slot 15''" cut sketch "草图16 (3)" along normal blind 4 bodies 32 in component "RS_RemovableGrate"
ref_plane "工作平面17" through (0, 0, 36) normal (0, 0, 1) x (1, 0, 0) in component "RS_RemovableGrate"
sketch "草图17 (3)" plane through (0, 0, 36) normal (0, 0, 1) x (1, 0, 0) in component "RS_RemovableGrate"
  line L0 (772.3, 224) -> (777.3, 224)
  line L1 (777.3, 224) -> (777.3, 240)
  line L2 (777.3, 240) -> (772.3, 240)
  line L3 (772.3, 240) -> (772.3, 224)
  dimension "d1866" = 772.3
  dimension "d1867" = 224
  dimension "d1868" = 5
  dimension "d1869" = 16
  constraint horizontal L0
  constraint vertical L1
  constraint horizontal L2
  constraint vertical L3
  measures "d1866" horizontal distance of origin L0.start
  measures "d1867" vertical distance of origin L0.start
  measures "d1868" horizontal distance of L0.start L0.end
  measures "d1869" vertical distance of L0.end L1.end
extrude "Finger lift notch'''''" cut sketch "草图17 (3)" along normal blind 4 bodies 32 in component "RS_RemovableGrate"
ref_plane "工作平面1" through (0, 0, 0) normal (0, 0, 1) x (1, 0, 0) in component "RS_Foot_00"
sketch "草图1 (33)" plane through (0, 0, 0) normal (0, 0, 1) x (1, 0, 0) in component "RS_Foot_00"
  line L0 (841, 145) -> (857, 145)
  line L1 (857, 145) -> (857, 161)
  line L2 (857, 161) -> (841, 161)
  line L3 (841, 161) -> (841, 145)
  dimension "d1874" = 841
  dimension "d1875" = 145
  dimension "d1876" = 16
  dimension "d1877" = 16
  constraint horizontal L0
  constraint vertical L1
  constraint horizontal L2
  constraint vertical L3
  measures "d1874" horizontal distance of origin L0.start
  measures "d1875" vertical distance of origin L0.start
  measures "d1876" horizontal distance of L0.start L0.end
  measures "d1877" vertical distance of L0.end L1.end
extrude "Foot base''''''''''''''''''''" add sketch "草图1 (33)" along normal blind 20 separate body makes body 33 in component "RS_Foot_00"
ref_plane "工作平面2" through (0, 0, 20) normal (0, 0, 1) x (1, 0, 0) in component "RS_Foot_00"
sketch "草图2 (33)" plane through (0, 0, 20) normal (0, 0, 1) x (1, 0, 0) in component "RS_Foot_00"
  line L0 (845, 149) -> (853, 149)
  line L1 (853, 149) -> (853, 157)
  line L2 (853, 157) -> (845, 157)
  line L3 (845, 157) -> (845, 149)
  dimension "d1882" = 845
  dimension "d1883" = 149
  dimension "d1884" = 8
  dimension "d1885" = 8
  constraint horizontal L0
  constraint vertical L1
  constraint horizontal L2
  constraint vertical L3
  measures "d1882" horizontal distance of origin L0.start
  measures "d1883" vertical distance of origin L0.start
  measures "d1884" horizontal distance of L0.start L0.end
  measures "d1885" vertical distance of L0.end L1.end
extrude "Locating peg''''''''''''''''''''" add sketch "草图2 (33)" along normal blind 1.5 bodies 33 in component "RS_Foot_00"
ref_plane "工作平面1" through (0, 0, 0) normal (0, 0, 1) x (1, 0, 0) in component "RS_Foot_01"
sketch "草图1 (34)" plane through (0, 0, 0) normal (0, 0, 1) x (1, 0, 0) in component "RS_Foot_01"
  line L0 (779, 145) -> (795, 145)
  line L1 (795, 145) -> (795, 161)
  line L2 (795, 161) -> (779, 161)
  line L3 (779, 161) -> (779, 145)
  dimension "d1890" = 779
  dimension "d1891" = 145
  dimension "d1892" = 16
  dimension "d1893" = 16
  constraint horizontal L0
  constraint vertical L1
  constraint horizontal L2
  constraint vertical L3
  measures "d1890" horizontal distance of origin L0.start
  measures "d1891" vertical distance of origin L0.start
  measures "d1892" horizontal distance of L0.start L0.end
  measures "d1893" vertical distance of L0.end L1.end
extrude "Foot base'''''''''''''''''''''" add sketch "草图1 (34)" along normal blind 20 separate body makes body 34 in component "RS_Foot_01"
ref_plane "工作平面2" through (0, 0, 20) normal (0, 0, 1) x (1, 0, 0) in component "RS_Foot_01"
sketch "草图2 (34)" plane through (0, 0, 20) normal (0, 0, 1) x (1, 0, 0) in component "RS_Foot_01"
  line L0 (783, 149) -> (791, 149)
  line L1 (791, 149) -> (791, 157)
  line L2 (791, 157) -> (783, 157)
  line L3 (783, 157) -> (783, 149)
  dimension "d1898" = 783
  dimension "d1899" = 149
  dimension "d1900" = 8
  dimension "d1901" = 8
  constraint horizontal L0
  constraint vertical L1
  constraint horizontal L2
  constraint vertical L3
  measures "d1898" horizontal distance of origin L0.start
  measures "d1899" vertical distance of origin L0.start
  measures "d1900" horizontal distance of L0.start L0.end
  measures "d1901" vertical distance of L0.end L1.end
extrude "Locating peg'''''''''''''''''''''" add sketch "草图2 (34)" along normal blind 1.5 bodies 34 in component "RS_Foot_01"
ref_plane "工作平面1" through (0, 0, 0) normal (0, 0, 1) x (1, 0, 0) in component "RS_Foot_10"
sketch "草图1 (35)" plane through (0, 0, 0) normal (0, 0, 1) x (1, 0, 0) in component "RS_Foot_10"
  line L0 (841, 303) -> (857, 303)
  line L1 (857, 303) -> (857, 319)
  line L2 (857, 319) -> (841, 319)
  line L3 (841, 319) -> (841, 303)
  dimension "d1906" = 841
  dimension "d1907" = 303
  dimension "d1908" = 16
  dimension "d1909" = 16
  constraint horizontal L0
  constraint vertical L1
  constraint horizontal L2
  constraint vertical L3
  measures "d1906" horizontal distance of origin L0.start
  measures "d1907" vertical distance of origin L0.start
  measures "d1908" horizontal distance of L0.start L0.end
  measures "d1909" vertical distance of L0.end L1.end
extrude "Foot base''''''''''''''''''''''" add sketch "草图1 (35)" along normal blind 20 separate body makes body 35 in component "RS_Foot_10"
ref_plane "工作平面2" through (0, 0, 20) normal (0, 0, 1) x (1, 0, 0) in component "RS_Foot_10"
sketch "草图2 (35)" plane through (0, 0, 20) normal (0, 0, 1) x (1, 0, 0) in component "RS_Foot_10"
  line L0 (845, 307) -> (853, 307)
  line L1 (853, 307) -> (853, 315)
  line L2 (853, 315) -> (845, 315)
  line L3 (845, 315) -> (845, 307)
  dimension "d1914" = 845
  dimension "d1915" = 307
  dimension "d1916" = 8
  dimension "d1917" = 8
  constraint horizontal L0
  constraint vertical L1
  constraint horizontal L2
  constraint vertical L3
  measures "d1914" horizontal distance of origin L0.start
  measures "d1915" vertical distance of origin L0.start
  measures "d1916" horizontal distance of L0.start L0.end
  measures "d1917" vertical distance of L0.end L1.end
extrude "Locating peg''''''''''''''''''''''" add sketch "草图2 (35)" along normal blind 1.5 bodies 35 in component "RS_Foot_10"
ref_plane "工作平面1" through (0, 0, 0) normal (0, 0, 1) x (1, 0, 0) in component "RS_Foot_11"
sketch "草图1 (36)" plane through (0, 0, 0) normal (0, 0, 1) x (1, 0, 0) in component "RS_Foot_11"
  line L0 (779, 303) -> (795, 303)
  line L1 (795, 303) -> (795, 319)
  line L2 (795, 319) -> (779, 319)
  line L3 (779, 319) -> (779, 303)
  dimension "d1922" = 779
  dimension "d1923" = 303
  dimension "d1924" = 16
  dimension "d1925" = 16
  constraint horizontal L0
  constraint vertical L1
  constraint horizontal L2
  constraint vertical L3
  measures "d1922" horizontal distance of origin L0.start
  measures "d1923" vertical distance of origin L0.start
  measures "d1924" horizontal distance of L0.start L0.end
  measures "d1925" vertical distance of L0.end L1.end
extrude "Foot base'''''''''''''''''''''''" add sketch "草图1 (36)" along normal blind 20 separate body makes body 36 in component "RS_Foot_11"
ref_plane "工作平面2" through (0, 0, 20) normal (0, 0, 1) x (1, 0, 0) in component "RS_Foot_11"
sketch "草图2 (36)" plane through (0, 0, 20) normal (0, 0, 1) x (1, 0, 0) in component "RS_Foot_11"
  line L0 (783, 307) -> (791, 307)
  line L1 (791, 307) -> (791, 315)
  line L2 (791, 315) -> (783, 315)
  line L3 (783, 315) -> (783, 307)
  dimension "d1930" = 783
  dimension "d1931" = 307
  dimension "d1932" = 8
  dimension "d1933" = 8
  constraint horizontal L0
  constraint vertical L1
  constraint horizontal L2
  constraint vertical L3
  measures "d1930" horizontal distance of origin L0.start
  measures "d1931" vertical distance of origin L0.start
  measures "d1932" horizontal distance of L0.start L0.end
  measures "d1933" vertical distance of L0.end L1.end
extrude "Locating peg'''''''''''''''''''''''" add sketch "草图2 (36)" along normal blind 1.5 bodies 36 in component "RS_Foot_11"
ref_plane "工作平面1" through (0, 0, 125) normal (0, 0, 1) x (1, 0, 0) in component "Tower_Integrated"
sketch "草图1 (37)" plane through (0, 0, 125) normal (0, 0, 1) x (1, 0, 0) in component "Tower_Integrated"
  line L0 (50, 50) -> (230, 50)
  line L1 (230, 50) -> (230, 140)
  line L2 (230, 140) -> (50, 140)
  line L3 (50, 140) -> (50, 50)
  dimension "d1938" = 50
  dimension "d1939" = 50
  dimension "d1940" = 180
  dimension "d1941" = 90
  constraint horizontal L0
  constraint vertical L1
  constraint horizontal L2
  constraint vertical L3
  measures "d1938" horizontal distance of origin L0.start
  measures "d1939" vertical distance of origin L0.start
  measures "d1940" horizontal distance of L0.start L0.end
  measures "d1941" vertical distance of L0.end L1.end